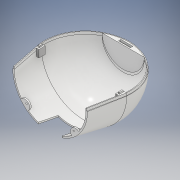
# Autodesk Inventor part: trasera
Saved by Autodesk Inventor 2017 (Build 210142000, 142)
## iProperties
Part Number: trasera
Material: Genérico
Document SubType Name: Modeling
Designer: Roberto
Density: 1 g/cm^3
Appearance: Valor por defecto
Author: Roberto
Autodesk Inventor part; units mm, degrees
ref_plane "YZ Plane" through (0, 0, 0) normal (1, 0, 0) x (0, 1, 0)
ref_plane "XZ Plane" through (0, 0, 0) normal (0, 1, 0) x (-1, 0, 0)
ref_plane "XY Plane" through (0, 0, 0) normal (0, 0, 1) x (1, 0, 0)
sketch "Boceto1" plane through (0, 0, 0) normal (0, 0, 1) x (1, 0, 0)
  line L0 (0, 0) -> (0.3056, 0)
  line L1 (-0.9959, 6.6959) -> (0.3056, 0)
  line L2 (-1.2332, 6.6387) -> (0, 0)
  arc A0 (3.3399, 14.6949) -> (-0.9959, 6.6959) centre (7.0639, 7.5017) ccw
  arc A1 (3.2285, 14.9096) -> (-1.2332, 6.6387) centre (7.0639, 7.5017) ccw
  line L3 (0, 0) -> (15, 0)
  line L4 (7.5, 15.7708) -> (7.5, 16.0128)
  arc A2 (7.5, 15.7708) -> (3.2727, 14.6597) centre (7.7745, 6.1292) ccw
  arc A3 (7.5, 16.0128) -> (3.2285, 14.9096) centre (7.7745, 6.1292) ccw
  line L5 (0, 0) -> (0.3056, 0)
  line L6 (0.3056, 0) -> (-0.9959, 6.6959)
  line L7 (-1.2332, 6.6387) -> (0, 0)
  line L8 (-1.2332, 6.6387) -> (-0.9959, 6.6959)
  line L9 (7.5, 16.0128) -> (7.5, 15.7708)
  dimension "d0" = 15
  constraints: 20 end point, 11 point on circle, 4 centre point, 3 collinear, 2 coincident, 2 horizontal, 1 perpendicular, 1 vertical
  measures "d0" distance of L0.start L3.end
revolve "Revolución1" add sketch "Boceto1" angle 180 about axis through (7.5, 15.7708, 0) along (0, -1, 0)
sketch "Boceto2" plane through (7.0639, 7.5017, 0) normal (0, 0, 1) x (0.8801071, -0.4747751, 0)
  line L0 (-2.3864, -9.811) -> (-6.7109, -4.5358) projected
  arc A0 (-6.7351, 4.4998) -> (-6.7109, -4.5358) centre (0, 0) ccw projected
  line L1 (8.2437, 3.5315) -> (10.2773, -2.9795) projected
  arc A1 (0.7059, 8.5139) -> (-3.5421, 7.4847) centre (0.7939, -1.1312) ccw projected
  arc A2 (-3.5421, 7.4847) -> (-6.7351, 4.4998) centre (1.277, -0.8706) ccw projected
  arc A3 (8.2437, 3.5315) -> (0.7059, 8.5139) centre (0.7676, 0.4141) ccw projected
  line L2 (-2.5209, -9.8835) -> (-6.8313, -4.6256)
  arc A4 (-6.8598, 4.5833) -> (-6.8313, -4.6256) centre (0, 0) ccw
  arc A5 (-3.6134, 7.6168) -> (-6.8598, 4.5833) centre (1.277, -0.8706) ccw
  arc A6 (0.7046, 8.6639) -> (-3.6134, 7.6168) centre (0.7939, -1.1312) ccw
  arc A7 (8.3848, 3.5828) -> (0.7046, 8.6639) centre (0.7676, 0.4141) ccw
  line L3 (8.3848, 3.5828) -> (10.4118, -2.907)
  line L4 (10.2773, -2.9795) -> (10.4118, -2.907)
  line L5 (10.2773, -2.9795) -> (10.5462, -2.8344) projected
  line L6 (-2.3864, -9.811) -> (-2.5209, -9.8835)
  line L7 (-2.6554, -9.9561) -> (-2.3864, -9.811) projected
  dimension "d2" = 0.15
  constraints: 8 end point, 8 point on circle, 4 centre point, 4 midpoint, 3 other
  measures "d2" radial gap between concentric circles of A3 A7
extrude "Extrusión1" add sketch "Boceto2" along normal blind 0.5
sketch "Boceto3" plane through (7.5, 0, 0) normal (0, -1, 0) x (1, 0, 0)
  arc A0 (-7.1944, 0) -> (7.1944, 0) centre (0, 0) ccw projected
  arc A1 (-7.5, 0) -> (7.5, 0) centre (0, 0) ccw projected
  line L0 (-4.2273, 0) -> (0, 0) projected
  line L1 (7.1944, 0) -> (7.1944, 0.5) projected
  line L2 (0, 0) -> (4.2273, 0) projected
  arc A2 (5.9447, -4.5728) -> (4.5728, -5.9447) centre (5.0872, -5.0872) ccw
  arc A3 (-4.5728, -5.9447) -> (-5.9447, -4.5728) centre (-5.0872, -5.0872) ccw
  line L3 (-5.9447, -4.5728) -> (-4.5728, -5.9447)
  line L4 (4.5728, -5.9447) -> (5.9447, -4.5728)
  dimension "d5" = 2
  constraints: 9 point on circle, 4 end point, 2 centre point
  measures "d5" diameter of A2
extrude "Extrusión2" add sketch "Boceto3" against normal blind 0.3 contours A3 A0 | A0 A3 L3 | A2 A0 | A0 A2 L4
sketch "Boceto4" plane through (7.5, 0, 0) normal (0, -1, 0) x (1, 0, 0)
  arc A0 (-4.3327, -5.7435) -> (-5.7435, -4.3327) centre (-5.0872, -5.0872) ccw projected
  arc A1 (5.7435, -4.3327) -> (4.3327, -5.7435) centre (5.0872, -5.0872) ccw projected
  circle A2 centre (-4.7337, -4.7337) radius 0.15
  circle A3 centre (4.7337, -4.7337) radius 0.15
  point P0 (-7.5, 0)
  dimension "d8" = 0.3
  dimension "d9" = 0.3
  constraints: 2 centre point
  measures "d8" diameter of A2
  measures "d9" diameter of A3
extrude "Extrusión3" cut sketch "Boceto4" against normal blind 0.3
sketch "Boceto6" plane through (7.0639, 7.5017, 0) normal (0, 0, 1) x (0.8801071, -0.4747751, 0)
  line L0 (0.1322, -8.4523) -> (7.7586, -4.3382) projected
  line L1 (-6.7351, 4.4998) -> (0.7059, 8.5139) projected
  line L2 (3.9454, -6.3953) -> (1.8332, -7.5347)
  line L3 (1.8332, -7.5347) -> (-0.0659, -4.0143)
  line L4 (-0.0659, -4.0143) -> (4.1586, -1.7354)
  line L5 (4.1586, -1.7354) -> (6.0577, -5.2558)
  line L6 (6.0577, -5.2558) -> (3.9454, -6.3953)
  point P0 (-2.6554, -9.9561)
  dimension "d14" = 2.4
  dimension "d15" = 4
  dimension "d16" = 4.8
  dimension "d17" = 4
  constraints: 10 end point, 2 perpendicular, 2 point on line, 1 midpoint
  measures "d14" distance of L2.start L2.end
  measures "d15" distance of L2.end L3.end
  measures "d16" distance of L3.end L4.end
  measures "d17" distance of L4.end L5.end
extrude "Extrusión4" cut sketch "Boceto6" against normal blind 30
sketch "Boceto7" plane through (7.0639, 7.5017, 0.5) normal (0, 0, 1) x (0.8801071, -0.4747751, 0)
  arc A0 (-3.5421, 7.4847) -> (-6.7351, 4.4998) centre (1.277, -0.8706) ccw projected
  line L0 (-6.7351, 4.4998) -> (0.7059, 8.5139) projected
  arc A1 (0.7059, 8.5139) -> (-3.5421, 7.4847) centre (0.7939, -1.1312) ccw projected
  line L1 (-3.5421, 7.4847) -> (-3.0146, 6.5069)
  line L2 (-3.0146, 6.5069) -> (-6.7351, 4.4998)
  arc A2 (-3.5421, 7.4847) -> (-6.7351, 4.4998) centre (1.277, -0.8706) ccw
  point P0 (-2.6554, -9.9561)
  constraints: 4 end point, 2 concentric, 2 point on circle, 1 centre point, 1 midpoint
revolve "Revolución2" add sketch "Boceto7" angle 180 about axis through (7.5, 15.7708, 0.5) along (0, -1, 0) contours L1 L0 A0
sketch "Boceto8" plane through (3.2727, 14.6597, 0.5) normal (0, 0, 1) x (1, 0, 0)
  line L0 (-4.2686, -7.9638) -> (-3.4686, -7.9638)
  line L1 (-4.2686, -7.9638) -> (-4.0257, -9.2138)
  line L2 (1.8273, -10.6597) -> (6.6273, -10.6597) projected
  line L3 (12.7233, -7.9638) -> (11.9233, -7.9638)
  line L4 (12.7233, -7.9638) -> (12.4317, -9.4638)
  line L5 (-3.4686, -9.2138) -> (-4.0257, -9.2138)
  line L6 (-3.4686, -9.2138) -> (-3.4686, -7.9638)
  line L7 (11.9233, -9.2138) -> (12.4803, -9.2138)
  line L8 (11.4217, -14.6597) -> (12.4317, -9.4638)
  line L9 (12.4803, -9.2138) -> (12.7233, -7.9638)
  line L10 (11.9233, -9.2138) -> (11.9233, -7.9638)
  point P0 (-3.2727, -14.6597)
  dimension "d21" = 0.8
  constraints: 20 end point, 2 vertical, 1 horizontal, 1 point on line
  measures "d21" distance of L0.start L0.end
extrude "Extrusión5" add sketch "Boceto8" against normal blind 1.5
sketch "Boceto9" plane through (3.2727, 14.6597, 0.5) normal (0, 0, 1) x (1, 0, 0)
  line L0 (0, 0) -> (8.4546, 0) projected
  line L1 (4.2273, 0.25) -> (5.4273, 0.2499)
  line L2 (-0.0441, 0.2499) -> (8.4988, 0.2499) projected
  line L3 (5.4273, 0.2499) -> (5.4274, 0.7499)
  line L4 (5.4274, 0.7499) -> (3.0274, 0.7501)
  line L5 (3.0274, 0.7501) -> (3.0273, 0.2499)
  line L6 (4.2273, 0.25) -> (3.0273, 0.2499)
  point P0 (-3.2727, -14.6597)
  dimension "d26" = 1.2
  dimension "d27" = 0.5
  dimension "d28" = 2.4
  constraints: 10 end point, 3 perpendicular, 2 point on line
  measures "d26" distance of L1.start L1.end
  measures "d27" distance of L1.end L3.end
  measures "d28" distance of L3.end L4.end
extrude "Extrusión6" cut sketch "Boceto9" against normal blind 0.4
sketch "Boceto10" plane through (7.0639, 7.5017, 0.5) normal (0, 0, 1) x (0.8801071, -0.4747751, 0)
  line L0 (-6.7109, -4.5358) -> (-6.0069, -4.156) projected
  line L1 (-5.2947, -5.4761) -> (-6.0069, -4.156) projected
  line L2 (-6.3272, -4.6128) -> (-6.1082, -4.4947)
  line L3 (-6.1082, -4.4947) -> (-5.8233, -5.0228)
  line L4 (4.1586, -1.7354) -> (-0.0659, -4.0143) projected
  line L5 (2.0463, -2.8748) -> (1.0275, -0.9862)
  line L6 (7.5396, 3.1517) -> (8.2437, 3.5315)
  line L7 (8.2518, 1.8315) -> (7.5396, 3.1517)
  line L8 (8.0973, 3.1685) -> (7.8784, 3.0504)
  line L9 (7.8784, 3.0504) -> (8.1632, 2.5223)
  line L10 (8.4297, 2.5524) -> (8.0973, 3.1685)
  line L11 (8.2107, 2.4343) -> (8.4297, 2.5524)
  line L12 (8.2107, 2.4343) -> (7.8784, 3.0504)
  line L13 (-5.7758, -5.1108) -> (-5.9948, -5.2289)
  line L14 (-5.9948, -5.2289) -> (-6.3272, -4.6128)
  line L15 (-5.7758, -5.1108) -> (-6.1082, -4.4947)
  point P0 (-2.6554, -9.9561)
  point P1 (-5.6809, -5.2868)
  point P2 (8.3057, 2.2583)
  dimension "d33" = 0.6
  dimension "d38" = 0.25
  dimension "d39" = 0.25
  constraints: 26 end point, 7 symmetric about line, 4 perpendicular, 2 point on line, 1 collinear, 1 midpoint
  measures "d33" distance of L2.end L3.end
  measures "d38" distance between parallel lines of L0 L2
  measures "d39" distance between parallel lines of L1 L3
extrude "Extrusión7" add sketch "Boceto10" along normal blind 0.3
